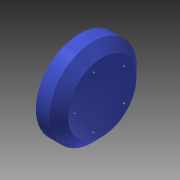
# Autodesk Inventor part: tool_2
Saved by Autodesk Inventor 2015 (Build 190159000, 159)
## iProperties
Created: 2015-12-22
Part Number: tool_2
Material: ABS プラスチック
Document SubType Name: Modeling
Designer: Ryo
Density: 1.06 g/cm^3
Appearance: 滑らか - 白
Author: Ryo
Autodesk Inventor part; units mm, degrees
ref_plane "YZ Plane" through (0, 0, 0) normal (1, 0, 0) x (0, 1, 0)
ref_plane "XZ Plane" through (0, 0, 0) normal (0, 1, 0) x (-1, 0, 0)
ref_plane "XY Plane" through (0, 0, 0) normal (0, 0, 1) x (1, 0, 0)
sketch "スケッチ1" plane through (0, 0, 0) normal (1, 0, 0) x (0, 1, 0)
  circle A0 centre (0, 0) radius 48
  dimension "d0" = 96
  constraints: 1 centre point, 1 coincident
  measures "d0" diameter of A0
extrude "押し出し1" add sketch "スケッチ1" along normal blind 17
sketch "スケッチ2" plane through (17, 0, 0) normal (1, 0, 0) x (0, 0, -1)
  circle A0 centre (0, 0) radius 48
  constraints: 1 centre point, 1 coincident
extrude "押し出し2" add sketch "スケッチ2" along normal blind 10
chamfer "面取り1" distance 10.5 distance2 10 1 edges at (27, 0, 48) measured on face at (27, 0, 47.5)
sketch "スケッチ3" plane through (0, 0, 0) normal (-1, 0, 0) x (0, 0, 1)
  circle A0 centre (0, 0) radius 40
  dimension "d8" = 80
  constraints: 1 centre point, 1 coincident
  measures "d8" diameter of A0
extrude "押し出し3" cut sketch "スケッチ3" against normal blind 8
chamfer "面取り2" distance 4 distance2 2 1 edges at (0, -48, 0) measured on face at (0, -47.5, 0)
fillet "フィレット1" radius 2 1 edges at (0, 0, -40)
fillet "フィレット2" radius 2 1 edges at (8, 0, -40)
sketch "スケッチ4" plane through (27, 0, 0) normal (1, 0, 0) x (0, 0, -1)
  circle A0 centre (0, -30) radius 1.5
  circle A1 centre (28.5317, -9.2705) radius 1.5
  circle A2 centre (17.6336, 24.2705) radius 1.5
  circle A3 centre (-17.6336, 24.2705) radius 1.5
  circle A4 centre (-28.5317, -9.2705) radius 1.5
  point P0 (0, 0)
  dimension "d16" = 3
  dimension "d17" = 30
  dimension "d20" = 360
  constraints: 5 centre point, 11 other
  measures "d16" diameter of A0
  measures "d17" distance of point (0, 0) A0.centre
extrude "押し出し4" cut sketch "スケッチ4" against normal blind 8
thread "ねじ1" size "M3x0.5" class "6H" standard "ANSI Metric M Profile" full length
thread "ねじ2" size "M3x0.5" class "6H" standard "ANSI Metric M Profile" full length
thread "ねじ3" size "M3x0.5" class "6H" standard "ANSI Metric M Profile" full length
thread "ねじ4" size "M3x0.5" class "6H" standard "ANSI Metric M Profile" full length
thread "ねじ5" size "M3x0.5" class "6H" standard "ANSI Metric M Profile" full length
